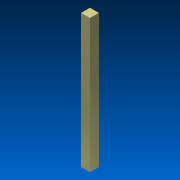
# Autodesk Inventor part: GoPro Hero 3 HDMI Pin
Saved by Autodesk Inventor 2015 (Build 190159000, 159)
## iProperties
Created: 2013-02-18
Project: GoPro Hero 3 HD Camera
Material: Copper
Description: GoPro Hero 3 HDMI Pin
Document SubType Name: Modeling
Designer: sdarley
Density: 1 g/cm^3
Appearance: Nickel
Title: GoPro Hero 3 HDMI Pin
Author: sdarley
Revision Number: 1
Autodesk Inventor part; units mm, degrees
ref_plane "YZ Plane" through (0, 0, 0) normal (1, 0, 0) x (0, 1, 0)
ref_plane "XZ Plane" through (0, 0, 0) normal (0, 1, 0) x (-1, 0, 0)
ref_plane "XY Plane" through (0, 0, 0) normal (0, 0, 1) x (1, 0, 0)
sketch "Sketch1" plane through (0, 0, 0) normal (0, 0, 1) x (1, 0, 0)
  line L0 (0.1, -0.1) -> (-0.1, -0.1)
  line L1 (-0.1, -0.1) -> (-0.1, 0.1)
  line L2 (-0.1, 0.1) -> (0.1, 0.1)
  line L3 (0.1, 0.1) -> (0.1, -0.1)
  line L4 (0.1, -0.1) -> (-0.1, 0.1) construction
  line L5 (-0.1, -0.1) -> (0.1, 0.1) construction
  point P0 (0, 0)
  dimension "d0" = 0.2
  dimension "d1" = 0.2
  constraints: 12 end point, 2 midpoint, 2 parallel, 1 horizontal, 1 perpendicular
  measures "d0" distance of L1.end L2.end
  measures "d1" distance of L0.end L1.end
extrude "Extrusion1" add sketch "Sketch1" along normal blind 3
equation "\"d0\" = d1"
body "Solid1"
